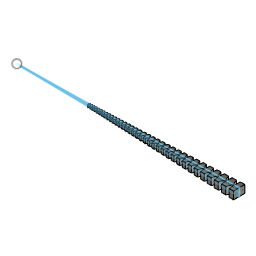
spiral arm 2d v1 (Autodesk Fusion 360 design; units mm, degrees)
Autodesk Fusion 360 part; units mm, degrees
note: some values were not read from the file. Chosen so that the rebuilt part matches the saved one: which bodies a step acts on; which face or edge a step refers to.
sketch "Sketch1" plane through (0, 0, 0) normal (0, 0, 1) x (1, 0, 0)
  line L0 (0, 0) -> (0.1753, 1.5)
  line L1 (0.1753, 1.5) -> (1.3453, 1.5)
  line L2 (1.3453, 1.5) -> (1.9923, 0)
  line L3 (2.9923, 0) -> (3.1764, 1.575)
  line L4 (3.1764, 1.575) -> (4.4049, 1.575)
  line L5 (4.4049, 1.575) -> (5.0843, 0)
  line L6 (6.0843, 0) -> (6.2776, 1.6538)
  line L7 (6.2776, 1.6538) -> (7.5675, 1.6538)
  line L8 (7.5675, 1.6538) -> (8.2809, 0)
  line L9 (9.2809, 0) -> (9.4838, 1.7364)
  line L10 (9.4838, 1.7364) -> (10.8382, 1.7364)
  line L11 (10.8382, 1.7364) -> (11.5872, 0)
  line L12 (12.5872, 0) -> (12.8003, 1.8233)
  line L13 (12.8003, 1.8233) -> (14.2225, 1.8233)
  line L14 (14.2225, 1.8233) -> (15.009, 0)
  line L15 (16.009, 0) -> (16.2327, 1.9144)
  line L16 (16.2327, 1.9144) -> (17.7259, 1.9144)
  line L17 (17.7259, 1.9144) -> (18.5517, 0)
  line L18 (19.5517, 0) -> (19.7867, 2.0101)
  line L19 (19.7867, 2.0101) -> (21.3546, 2.0101)
  line L20 (21.3546, 2.0101) -> (22.2217, 0)
  line L21 (23.2217, 0) -> (23.4683, 2.1107)
  line L22 (23.4683, 2.1107) -> (25.1147, 2.1107)
  line L23 (25.1147, 2.1107) -> (26.0251, 0)
  line L24 (27.0251, 0) -> (27.2841, 2.2162)
  line L25 (27.2841, 2.2162) -> (29.0127, 2.2162)
  line L26 (29.0127, 2.2162) -> (29.9687, 0)
  line L27 (30.9687, 0) -> (31.2407, 2.327)
  line L28 (31.2407, 2.327) -> (33.0557, 2.327)
  line L29 (33.0557, 2.327) -> (34.0595, 0)
  line L30 (35.0595, 0) -> (35.345, 2.4433)
  line L31 (35.345, 2.4433) -> (37.2508, 2.4433)
  line L32 (37.2508, 2.4433) -> (38.3048, 0)
  line L33 (39.3048, 0) -> (39.6046, 2.5655)
  line L34 (39.6046, 2.5655) -> (41.6057, 2.5655)
  line L35 (41.6057, 2.5655) -> (42.7124, 0)
  line L36 (43.7124, 0) -> (44.0272, 2.6938)
  line L37 (44.0272, 2.6938) -> (46.1284, 2.6938)
  line L38 (46.1284, 2.6938) -> (47.2903, 0)
  line L39 (48.2903, 0) -> (48.6209, 2.8285)
  line L40 (48.6209, 2.8285) -> (50.8271, 2.8285)
  line L41 (50.8271, 2.8285) -> (52.0472, 0)
  line L42 (53.0472, 0) -> (53.3943, 2.9699)
  line L43 (53.3943, 2.9699) -> (55.7108, 2.9699)
  line L44 (55.7108, 2.9699) -> (56.9919, 0)
  line L45 (57.9919, 0) -> (58.3564, 3.1184)
  line L46 (58.3564, 3.1184) -> (60.7887, 3.1184)
  line L47 (60.7887, 3.1184) -> (62.1338, 0)
  line L48 (63.1338, 0) -> (63.5165, 3.2743)
  line L49 (63.5165, 3.2743) -> (66.0705, 3.2743)
  line L50 (66.0705, 3.2743) -> (67.4829, 0)
  line L51 (68.4829, 0) -> (68.8847, 3.438)
  line L52 (68.8847, 3.438) -> (71.5663, 3.438)
  line L53 (71.5663, 3.438) -> (73.0494, 0)
  line L54 (74.0494, 0) -> (74.4713, 3.6099)
  line L55 (74.4713, 3.6099) -> (77.287, 3.6099)
  line L56 (77.287, 3.6099) -> (78.8442, 0)
  line L57 (79.8442, 0) -> (80.2872, 3.7904)
  line L58 (80.2872, 3.7904) -> (83.2437, 3.7904)
  line L59 (83.2437, 3.7904) -> (84.8787, 0)
  line L60 (85.8787, 0) -> (86.3439, 3.9799)
  line L61 (86.3439, 3.9799) -> (89.4482, 3.9799)
  line L62 (89.4482, 3.9799) -> (91.165, 0)
  line L63 (92.165, 0) -> (92.6534, 4.1789)
  line L64 (92.6534, 4.1789) -> (95.913, 4.1789)
  line L65 (95.913, 4.1789) -> (97.7156, 0)
  line L66 (98.7156, 0) -> (99.2284, 4.3879)
  line L67 (99.2284, 4.3879) -> (102.651, 4.3879)
  line L68 (102.651, 4.3879) -> (104.5437, 0)
  line L69 (105.5437, 0) -> (106.0822, 4.6073)
  line L70 (106.0822, 4.6073) -> (109.6759, 4.6073)
  line L71 (109.6759, 4.6073) -> (111.6632, 0)
  line L72 (112.6632, 0) -> (113.2286, 4.8376)
  line L73 (113.2286, 4.8376) -> (117.002, 4.8376)
  line L74 (117.002, 4.8376) -> (119.0887, 0)
  line L75 (120.0887, 0) -> (120.6824, 5.0795)
  line L76 (120.6824, 5.0795) -> (124.6444, 5.0795)
  line L77 (124.6444, 5.0795) -> (126.8355, 0)
  line L78 (127.8355, 0) -> (128.4589, 5.3335)
  line L79 (128.4589, 5.3335) -> (132.619, 5.3335)
  line L80 (132.619, 5.3335) -> (134.9196, 0)
  line L81 (135.9196, 0) -> (136.5742, 5.6002)
  line L82 (136.5742, 5.6002) -> (140.9423, 5.6002)
  line L83 (140.9423, 5.6002) -> (143.358, 0)
  line L84 (144.358, 0) -> (145.0452, 5.8802)
  line L85 (145.0452, 5.8802) -> (149.6318, 5.8802)
  line L86 (149.6318, 5.8802) -> (152.1682, 0)
  line L87 (153.1682, 0) -> (153.8898, 6.1742)
  line L88 (153.8898, 6.1742) -> (158.7057, 6.1742)
  line L89 (158.7057, 6.1742) -> (161.369, 0)
  line L90 (162.369, 0) -> (163.1266, 6.4829)
  line L91 (163.1266, 6.4829) -> (168.1833, 6.4829)
  line L92 (168.1833, 6.4829) -> (170.9798, 0)
  line L93 (171.9798, 0) -> (172.7753, 6.8071)
  line L94 (172.7753, 6.8071) -> (178.0848, 6.8071)
  line L95 (178.0848, 6.8071) -> (181.0211, 0)
  line L96 (182.0211, 0) -> (182.8564, 7.1474)
  line L97 (182.8564, 7.1474) -> (188.4314, 7.1474)
  line L98 (188.4314, 7.1474) -> (191.5145, 0)
  line L99 (192.5145, 0) -> (193.3916, 7.5048)
  line L100 (193.3916, 7.5048) -> (199.2453, 7.5048)
  line L101 (199.2453, 7.5048) -> (202.4826, 0)
  line L102 (203.4826, 0) -> (204.4035, 7.88)
  line L103 (204.4035, 7.88) -> (210.5499, 7.88)
  line L104 (210.5499, 7.88) -> (213.949, 0)
  line L105 (0, 0) -> (214.949, 0)
extrude "Extrude1" add sketch "Sketch1" along normal mid plane 40 makes body 1 at (185.1856, 0, 6.6667) makes body 2 at (149.5648, 0, 6.6667) makes body 3 at (116.9469, 0, 6.6667) makes body 4 at (89.4029, 0, 6.6667) makes body 5 at (66.0332, 0, 6.6667) makes body 6 at (44.905, 0, 6.6667) makes body 7 at (28.9875, 0, 6.6667) makes body 8 at (13.3945, 0, 6.6667) makes body 9 at (1.3282, 0, 6.6667) makes body 10 at (10.0497, 0, 6.6667) makes body 11 at (25.0906, 0, 6.6667) makes body 12 at (41.5765, 0, 6.6667) makes body 13 at (59.3725, 0, 6.6667) makes body 14 at (81.5224, 0, 6.6667) makes body 15 at (109.6234, 0, 6.6667) makes body 16 at (138.3991, 0, 6.6667) makes body 17 at (174.9935, 0, 6.6667) makes body 18 at (199.1599, 0, 6.6667) makes body 19 at (158.6354, 0, 6.6667) makes body 20 at (124.5866, 0, 6.6667) makes body 21 at (95.8654, 0, 6.6667) makes body 22 at (71.5272, 0, 6.6667) makes body 23 at (50.7949, 0, 6.6667) makes body 24 at (33.0292, 0, 6.6667) makes body 25 at (17.7041, 0, 6.6667) makes body 26 at (4.387, 0, 6.6667) makes body 27 at (6.8165, 0, 6.6667) makes body 28 at (21.3317, 0, 6.6667) makes body 29 at (36.1412, 0, 6.6667) makes body 30 at (55.677, 0, 6.6667) makes body 31 at (75.6476, 0, 6.6667) makes body 32 at (102.601, 0, 6.6667) makes body 33 at (132.5583, 0, 6.6667) makes body 34 at (165.2392, 0, 6.6667) makes body 35 at (210.4602, 0, 6.6667)
mirror "Mirror1" about plane through (203.4826, 0, 0) normal (0, -1, 0) of bodies 9 16 32 20 8 3 29 27 17 12 24 34 5 26 30 7 4 1 6 31 11 35 10 33 25 14 28 21 15 2 18 23 19 13 22 merged
sketch "Sketch3" plane through (0, 0, 0) normal (0, 1, 0) x (1, 0, 0)
  line L0 (210.5071, 0) -> (-100, 0)
  line L1 (-100, 0) -> (210.5071, -5.3668)
  line L2 (210.5071, -5.3668) -> (210.5071, 0)
  line L3 (-100, 0) -> (210.5071, 5.3668)
  line L4 (210.5071, 5.3668) -> (210.5071, 0)
  constraint horizontal L0
  constraint perpendicular L0 L2
  constraint symmetric L1.start L0 L3.start
  constraint symmetric L0 L1.end L3.end
sketch "Sketch4" plane through (210.5071, 0, 0) normal (1, 0, 0) x (0, 1, 0)
  line L0 (7.88, 5.3668) -> (-7.88, 5.3668)
  line L1 (-7.88, 5.3668) -> (-7.88, -5.3668)
  line L2 (-7.88, -5.3668) -> (7.88, -5.3668)
  circle A0 centre (5, 0) radius 0.25
  dimension "d7" = 0.5
  measures "d7" diameter of A0
sketch "Sketch5" plane through (0, 0, 0) normal (1, 0, 0) x (0, 1, 0)
  circle A0 centre (1, 0) radius 0.25
  dimension "d8" = 0.5
  measures "d8" diameter of A0
loft "Loft1" add profiles "Sketch4", "Sketch5" section 1 section 2 separate body makes body 70
mirror "Mirror2" about plane through (0, 0, 0) normal (0, 1, 0) of bodies 70 makes body 71
sketch "Sketch6" plane through (210.5071, 0, 0) normal (1, 0, 0) x (0, 1, 0)
  line L0 (10, 22) -> (-10, 22)
  line L1 (-10, 22) -> (-10, 17)
  line L2 (-10, 17) -> (10, 17)
  line L3 (10, 17) -> (10, 22)
  constraint horizontal L0
  constraint vertical L1
  constraint horizontal L2
  constraint vertical L3
extrude "Extrude3" add sketch "Sketch6" against normal blind 220 bodies 1 2 3 4 5 6 7 8 9 10 11 12 13 14 15 16 17 18 19 20 21 22 23 24 25 26 27 28 29 30 31 32 33 34 35
combine "Combine1" operation cut target body 1 tool bodies 70 71
extrude "Extrude4" cut sketch "Sketch3" along normal mid plane 60 keep common part bodies 1 makes body 72 at (210.5071, -1.6147, 3.643) makes body 73 at (131.7914, 1.7778, -4.0063) makes body 74 at (76.7268, 1.2033, -3.0545) makes body 75 at (36.8717, 0.8144, -2.3657) makes body 76 at (7.888, -0.9107, 1.3236) makes body 77 at (18.0928, 1.0638, -1.4417) makes body 78 at (50.3882, 0.9428, -2.5993) makes body 79 at (95.2645, 1.393, -3.3749) makes body 80 at (157.7476, 2.0581, -4.4549) makes body 81 at (177.0286, 2.269, -4.7881) makes body 82 at (108.9609, 1.5358, -3.6117) makes body 83 at (60.3048, 1.0395, -2.7707) makes body 84 at (25.5214, 1.1676, 1.5245) makes body 85 at (1.6393, 0.8186, -1.2511) makes body 86 at (29.4388, 1.2285, -1.5701) makes body 87 at (65.5624, 1.0914, -2.8616) makes body 88 at (116.2513, 1.6125, -3.7377) makes body 89 at (187.3223, 2.3825, -4.9661) makes body 90 at (148.7193, 1.9601, -4.2989) makes body 91 at (88.8306, 1.3266, -3.2637) makes body 92 at (45.7104, 0.8979, -2.5184) makes body 93 at (14.5761, 1.0035, -1.3987) makes body 94 at (11.175, 0.9556, -1.3604) makes body 95 at (41.2076, 0.8552, -2.4406) makes body 96 at (82.6555, 1.2635, -3.157) makes body 97 at (140.0733, 1.8667, -4.1494) makes body 98 at (198.0808, 2.5016, -5.152) makes body 99 at (123.8562, 1.6932, -3.8691) makes body 100 at (71.0329, 1.146, -2.9561) makes body 101 at (33.5013, 1.2939, -1.6179) makes body 102 at (4.7131, 0.8605, -1.2857) makes body 103 at (21.7408, 1.1148, 1.4826) makes body 104 at (55.25, 0.99, -2.6833) makes body 105 at (101.9701, 1.4626, -3.4908)
named bodies: "guide", "guide2"
